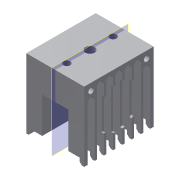
# Autodesk Inventor part: Part27
Saved by Autodesk Inventor 2016 (Build 200138000, 138)
## iProperties
Created: 2016-01-20
Part Number: Part27
Material: Aluminum 6061
Document SubType Name: Modeling
Designer: admin
Density: 2.71 g/cm^3
Appearance: Aluminum - Flat
Mass: 22.7069 g
Surface Area: 100.36 cm^2
Volume: 8.37892 cm^3
Author: admin
Autodesk Inventor part; units mm, degrees
ref_plane "YZ Plane" through (0, 0, 0) normal (1, 0, 0) x (0, 1, 0)
ref_plane "XZ Plane" through (0, 0, 0) normal (0, 1, 0) x (-1, 0, 0)
sketch "Sketch1" plane through (0, 0, 0) normal (0, 0, 1) x (1, 0, 0)
  circle A0 centre (0, 0) radius 4 projected
  circle A1 centre (0, -10) radius 1.5 projected
  circle A2 centre (0, 10) radius 1.5 projected
  line L0 (-5.5, -15) -> (5.5, -15) projected
  line L1 (5.5, -15) -> (5.5, 15) projected
  line L2 (5.5, 15) -> (-5.5, 15) projected
  line L3 (-5.5, 15) -> (-5.5, -15) projected
  point P0 (0, 0)
extrude "Extrusion1" add sketch "Sketch1" along normal blind 12
sketch "Sketch2" plane through (0, 0, 12) normal (0, 0, 1) x (1, 0, 0)
  line L0 (-5.5, 15) -> (-5.5, -15) projected
  line L1 (5.5, 15) -> (12.5, 15)
  line L2 (12.5, 15) -> (12.5, -15)
  line L3 (12.5, -15) -> (5.5, -15)
  line L4 (5.5, -15) -> (5.5, 15)
  line L5 (-5.5, 15) -> (-12.5, 15)
  line L6 (-12.5, 15) -> (-12.5, -15)
  line L7 (-12.5, -15) -> (-5.5, -15)
  line L8 (-5.5, -15) -> (-5.5, 15)
  dimension "d2" = 7
  dimension "d3" = 7
  constraints: 16 end point, 4 parallel, 2 horizontal, 2 perpendicular
  measures "d2" distance between parallel lines of L2 L4
  measures "d3" distance between parallel lines of L6 L0
extrude "Extrusion2" add sketch "Sketch2" against normal blind 30
sketch "Sketch4" plane through (0, 0, 12) normal (0, 0, 1) x (1, 0, 0)
  circle A0 centre (0, 0) radius 4 projected
  circle A1 centre (0, 0) radius 2.05
  dimension "d9" = 4.1
  constraints: 1 centre point, 1 coincident
  measures "d9" diameter of A1
extrude "Extrusion4" add sketch "Sketch4" against normal blind 1.5
sketch "Sketch5" plane through (-12.5, -15, 12) normal (-1, 0, 0) x (0, 0, 1)
  line L0 (0, 30) -> (0, 0) projected
  line L1 (0, 30) -> (-30, 30) projected
  line L2 (-30, 0) -> (-30, 30) projected
  line L3 (0, 0) -> (-30, 0) projected
  circle A0 centre (-27, 27) radius 1.5
  circle A1 centre (-3, 27) radius 1.2
  circle A2 centre (-27, 3) radius 1.5
  circle A3 centre (-3, 3) radius 1.2
  point P0 (-12, 15)
  dimension "d12" = 3
  dimension "d13" = 2.4
  dimension "d14" = 3
  dimension "d15" = 2.4
  dimension "d16" = 3
  dimension "d17" = 3
  dimension "d18" = 3
  dimension "d19" = 3
  dimension "d20" = 3
  dimension "d21" = 3
  dimension "d22" = 3
  dimension "d23" = 3
  constraints: 4 centre point
  measures "d12" diameter of A0
  measures "d13" diameter of A1
  measures "d14" diameter of A2
  measures "d15" diameter of A3
  measures "d16" distance from line of L2 A2.centre
  measures "d17" distance from line of L3 A2.centre
  measures "d18" distance from line of L3 A3.centre
  measures "d19" distance from line of L0 A3.centre
  measures "d20" distance from line of L0 A1.centre
  measures "d21" distance from line of L1 A1.centre
  measures "d22" distance from line of L1 A0.centre
  measures "d23" distance from line of L2 A0.centre
extrude "Extrusion5" cut sketch "Sketch5" against normal blind 7 contours A1 | A3
thread "Thread1" size "M3x0.5" class "6H" standard "ANSI Metric M Profile" full length
thread "Thread2" size "M3x0.5" class "6H" standard "ANSI Metric M Profile" full length
sketch "Sketch6" plane through (-12.5, -15, 12) normal (-1, 0, 0) x (0, 0, 1)
  circle A0 centre (-3, 27) radius 1.2 projected
  line L0 (0, 30) -> (0, 0) projected
  line L1 (0, 30) -> (-30, 30) projected
  line L2 (0, 0) -> (-30, 0) projected
  line L3 (-31, 27) -> (-7, 27) construction
  line L4 (-31, 28.5) -> (-7, 28.5)
  line L5 (-7, 25.5) -> (-31, 25.5)
  arc A1 (-31, 28.5) -> (-31, 25.5) centre (-31, 27) ccw
  arc A2 (-7, 25.5) -> (-7, 28.5) centre (-7, 27) ccw
  line L6 (-31, 3) -> (-7, 3) construction
  line L7 (-31, 1.5) -> (-7, 1.5)
  line L8 (-7, 4.5) -> (-31, 4.5)
  arc A3 (-31, 4.5) -> (-31, 1.5) centre (-31, 3) ccw
  arc A4 (-7, 1.5) -> (-7, 4.5) centre (-7, 3) ccw
  line L9 (-31, 23) -> (-3, 23) construction
  line L10 (-31, 21.5) -> (-3, 21.5)
  line L11 (-3, 24.5) -> (-31, 24.5)
  arc A5 (-31, 24.5) -> (-31, 21.5) centre (-31, 23) ccw
  arc A6 (-3, 21.5) -> (-3, 24.5) centre (-3, 23) ccw
  line L12 (-31, 19) -> (-3, 19) construction
  line L13 (-31, 17.5) -> (-3, 17.5)
  line L14 (-3, 20.5) -> (-31, 20.5)
  arc A7 (-31, 20.5) -> (-31, 17.5) centre (-31, 19) ccw
  arc A8 (-3, 17.5) -> (-3, 20.5) centre (-3, 19) ccw
  line L15 (-31, 11) -> (-3, 11) construction
  line L16 (-31, 9.5) -> (-3, 9.5)
  line L17 (-3, 12.5) -> (-31, 12.5)
  arc A9 (-31, 12.5) -> (-31, 9.5) centre (-31, 11) ccw
  arc A10 (-3, 9.5) -> (-3, 12.5) centre (-3, 11) ccw
  line L18 (-31, 7) -> (-3, 7) construction
  line L19 (-31, 5.5) -> (-3, 5.5)
  line L20 (-3, 8.5) -> (-31, 8.5)
  arc A11 (-31, 8.5) -> (-31, 5.5) centre (-31, 7) ccw
  arc A12 (-3, 5.5) -> (-3, 8.5) centre (-3, 7) ccw
  line L21 (-31, 15) -> (-3, 15) construction
  line L22 (-31, 13.5) -> (-3, 13.5)
  line L23 (-3, 16.5) -> (-31, 16.5)
  arc A13 (-31, 16.5) -> (-31, 13.5) centre (-31, 15) ccw
  arc A14 (-3, 13.5) -> (-3, 16.5) centre (-3, 15) ccw
  line L24 (-31, 23) -> (-31, 7)
  point P0 (-12, 15)
  point P1 (-19, 27)
  point P2 (-19, 3)
  point P3 (-17, 23)
  point P4 (-17, 19)
  point P5 (-17, 11)
  point P6 (-17, 7)
  point P7 (-17, 15)
  dimension "d34" = 1.5
  dimension "d35" = 4
  dimension "d37" = 1.5
  dimension "d38" = 3
  dimension "d39" = 3
  dimension "d40" = 3
  dimension "d41" = 3
  dimension "d42" = 3
  dimension "d43" = 1.5
  dimension "d44" = 1
  dimension "d45" = 1
  dimension "d46" = 1
  dimension "d47" = 1
  dimension "d48" = 3
  dimension "d49" = 3
  dimension "d51" = 1
  constraints: 58 end point, 28 point on circle, 28 tangent, 14 centre point, 14 parallel, 8 midpoint, 2 point on line, 1 perpendicular
  measures "d34" radius of A1
  measures "d35" distance of A0.centre L3.end
  measures "d37" distance between parallel lines of L1 L4
  measures "d38" diameter of A4
  measures "d39" diameter of A6
  measures "d40" diameter of A8
  measures "d41" diameter of A10
  measures "d42" diameter of A12
  measures "d43" distance between parallel lines of L2 L7
  measures "d44" distance between parallel lines of L19 L8
  measures "d45" distance between parallel lines of L16 L20
  measures "d46" distance between parallel lines of L5 L11
  measures "d47" distance between parallel lines of L10 L14
  measures "d48" diameter of A14
  measures "d49" distance from line of L0 L9.end
  measures "d51" distance between parallel lines of L17 L22
extrude "Extrusion6" cut sketch "Sketch6" against normal blind 6 contours L4 A2 L5 A1 | A3 L8 A4 L7 | A5 L11 A6 L10 | L20 A12 L19 A11 | L17 A10 L16 L24 | L24 A9 | L23 A14 L22 L24 | L24 A13 | L14 A8 L13 L24 | L24 A7
sketch "Sketch7" plane through (0, 0, -18) normal (0, 0, -1) x (-1, 0, 0)
  line L0 (12.5, 15) -> (5.5, 15) projected
  line L1 (5.5, 15) -> (5.5, -15) projected
  line L2 (5.5, -15) -> (12.5, -15) projected
  line L3 (12.5, -15) -> (12.5, 15) projected
  line L4 (10.5, -15) -> (10.5, 15)
  point P0 (0, 0)
  point P1 (9.8, -0.4092)
  dimension "d57" = 2
  constraints: 2 end point, 2 point on line
  measures "d57" distance between parallel lines of L3 L4
extrude "Extrusion7" cut sketch "Sketch7" against normal blind 2.5 contours L4 L2 L1 L0
ref_plane "Work Plane1" through (0, -15, 12) normal (-1, 0, 0) x (0, 0, 1)
sketch "Sketch9" plane through (-12.5, -15, 12) normal (-1, 0, 0) x (0, 0, 1)
  line L0 (0, 30) -> (0, 0) projected
  line L1 (0, 30) -> (-30, 30) projected
  circle A0 centre (-15, 15) radius 9
  point P0 (-7, 3)
  dimension "d88" = 18
  constraints: 1 centre point
  measures "d88" diameter of A0
extrude "Extrusion9" cut sketch "Sketch9" against normal blind 1
mirror "Mirror1" about plane through (0, -15, 12) normal (-1, 0, 0) of "Extrusion9", "Extrusion7", "Extrusion6", "Extrusion5"
chamfer "Chamfer1" distance 1 angle 45 16 edges at (-10.5, 14.25, -18) (-10.5, 10, -18) (-10.5, 6, -18) (-10.5, 2, -18) (-10.5, -2, -18) (-10.5, -6, -18) (-10.5, -10, -18) (-10.5, -14.25, -18) (10.5, 14.25, -18) (10.5, 10, -18) (10.5, 6, -18) (10.5, 2, -18) (10.5, -2, -18) (10.5, -6, -18) (10.5, -10, -18) (10.5, -14.25, -18)
sketch "Sketch11" plane through (-6.5, -15, 12) normal (-1, 0, 0) x (0, 0, 1)
  line L0 (-3, 5.5) -> (-27.5, 5.5) projected
  arc A0 (-3, 5.5) -> (-3, 8.5) centre (-3, 7) ccw projected
  line L1 (-27.5, 8.5) -> (-3, 8.5) projected
  line L2 (-27.5, 24.5) -> (-27.5, 21.5) projected
  line L3 (-3, 21.5) -> (-27.5, 21.5) projected
  arc A1 (-3, 21.5) -> (-3, 24.5) centre (-3, 23) ccw projected
  line L4 (-27.5, 24.5) -> (-3, 24.5) projected
  line L5 (-27.5, 28.5) -> (-27.5, 25.5) projected
  line L6 (-7, 25.5) -> (-27.5, 25.5) projected
  arc A2 (-7, 25.5) -> (-7, 28.5) centre (-7, 27) ccw projected
  line L7 (-27.5, 28.5) -> (-7, 28.5) projected
  line L8 (-27.5, 4.5) -> (-27.5, 1.5) projected
  line L9 (-7, 1.5) -> (-27.5, 1.5) projected
  arc A3 (-7, 1.5) -> (-7, 4.5) centre (-7, 3) ccw projected
  line L10 (-27.5, 4.5) -> (-7, 4.5) projected
  arc A4 (-10, 28.5) -> (-10, 25.5) centre (-10, 27) ccw
  arc A5 (-10, 24.5) -> (-10, 21.5) centre (-10, 23) ccw
  arc A6 (-10, 8.5) -> (-10, 5.5) centre (-10, 7) ccw
  arc A7 (-10, 4.5) -> (-10, 1.5) centre (-10, 3) ccw
  point P0 (-12, 15)
  dimension "d79" = 3
  constraints: 8 point on circle, 8 point on line, 4 centre point, 4 tangent
  measures "d79" distance of A2.centre A4.centre
extrude "Extrusion11" cut sketch "Sketch11" against normal blind 4 contours L0 A6 L1 A0 | L4 A1 L3 A5 | L7 A2 L6 A4 | L10 A3 L9 A7
sketch "Sketch12" plane through (-6.5, -15, 12) normal (-1, 0, 0) x (0, 0, 1)
  line L0 (-3, 9.5) -> (-27.5, 9.5) projected
  arc A0 (-3, 9.5) -> (-3, 12.5) centre (-3, 11) ccw projected
  line L1 (-27.5, 12.5) -> (-3, 12.5) projected
  line L2 (-27.5, 16.5) -> (-27.5, 13.5) projected
  line L3 (-3, 13.5) -> (-27.5, 13.5) projected
  arc A1 (-3, 13.5) -> (-3, 16.5) centre (-3, 15) ccw projected
  line L4 (-27.5, 16.5) -> (-3, 16.5) projected
  line L5 (-27.5, 20.5) -> (-27.5, 17.5) projected
  line L6 (-3, 17.5) -> (-27.5, 17.5) projected
  arc A2 (-3, 17.5) -> (-3, 20.5) centre (-3, 19) ccw projected
  line L7 (-27.5, 20.5) -> (-3, 20.5) projected
  arc A3 (-3, 21.5) -> (-3, 24.5) centre (-3, 23) ccw projected
  line L8 (-10, 24.5) -> (-3, 24.5) projected
  arc A4 (-10, 24.5) -> (-10, 21.5) centre (-10, 23) ccw projected
  line L9 (-3, 21.5) -> (-10, 21.5) projected
  arc A5 (-3, 5.5) -> (-3, 8.5) centre (-3, 7) ccw projected
  line L10 (-10, 8.5) -> (-3, 8.5) projected
  arc A6 (-10, 8.5) -> (-10, 5.5) centre (-10, 7) ccw projected
  line L11 (-3, 5.5) -> (-10, 5.5) projected
  arc A7 (-10, 12.5) -> (-10, 9.5) centre (-10, 11) ccw
  arc A8 (-10, 20.5) -> (-10, 17.5) centre (-10, 19) ccw
  arc A9 (-10, 16.5) -> (-10, 13.5) centre (-10, 15) ccw
  point P0 (-12, 15)
  constraints: 6 point on circle, 6 point on line, 3 centre point, 3 tangent
extrude "Extrusion12" cut sketch "Sketch12" against normal blind 2 contours L0 A7 L1 A0 | L4 A1 L3 A9 | L7 A2 L6 A8
mirror "Mirror2" about plane through (0, -15, 12) normal (-1, 0, 0) of "Extrusion11", "Extrusion12"
sketch "Sketch13" plane through (10.5, -15, -15.5) normal (0, 0, -1) x (-1, 0, 0)
  line L0 (5, 30) -> (5, 0) projected
  line L1 (4.85, 32.1879) -> (16.15, 32.1879)
  line L2 (16.15, 32.1879) -> (16.15, -3.2103)
  line L3 (16.15, -3.2103) -> (4.85, -3.2103)
  line L4 (4.85, -3.2103) -> (4.85, 32.1879)
  line L5 (16, 29) -> (16, -10) projected
  point P0 (10.5, 15)
  dimension "d84" = 0.15
  dimension "d85" = 0.15
  constraints: 8 end point, 2 parallel, 1 horizontal, 1 perpendicular
  measures "d84" distance between parallel lines of L0 L4
  measures "d85" distance between parallel lines of L2 L5
ref_plane "Work Plane2" through (-20.175, -20.3808, 0) normal (0, 0, 1) x (1, 0, 0)
extrude "Extrusion13" cut sketch "Sketch13" against normal up to surface (15.5 mm away)
fillet "Fillet2" radius 0.3 8 edges at (-12, 6.5, 3.2249) (-12, 6.5, -9.2249) (-12, -6.5, -9.2249) (-12, -6.5, 3.2249) (12, -6.5, -9.2249) (12, -6.5, 3.2249) (12, 6.5, 3.2249) (12, 6.5, -9.2249)
body "Solid1"
